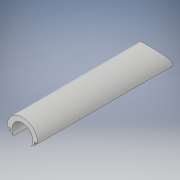
# Autodesk Inventor part: drone motor arm top
Saved by Autodesk Inventor 2019 (Build 230136000, 136)
## iProperties
Created: 2020-03-26
Part Number: drone motor arm top
Material: Generic
Document SubType Name: Modeling
Designer: Administrator
Density: 1 g/cm^3
Appearance: Default
Title: drone motor wrapper
Author: Administrator
Autodesk Inventor part; units mm, degrees
ref_plane "YZ Plane" through (0, 0, 0) normal (1, 0, 0) x (0, 1, 0)
ref_plane "Work Plane2" through (0.0017, -6.74, -2) normal (0, 1, 0) x (-1, 0, 0)
sketch "Sketch1" plane through (0.0017, -6.74, -2) normal (0, 1, 0) x (-1, 0, 0)
  line L0 (-2.7483, 0) -> (0, 0) construction
  line L1 (0, 0) -> (0.0017, 6)
  line L2 (1.7517, 6) -> (-1.7483, 6) construction
  arc A0 (-3.9294, 1.3826) -> (-4.2492, 3) centre (0.0008, 3) ccw construction
  arc A1 (-3.413, 0.4685) -> (3.4132, 0.4666) centre (0.0008, 3) ccw construction
  line L3 (5.1396, 2.9983) -> (6.2508, 2.9983)
  arc A2 (-6.2492, 3.0017) -> (6.2508, 2.9983) centre (0.0008, 3) ccw construction
  line L4 (5.7129, 2.1908) -> (5.1396, 2.1908) construction
  line L5 (5.1396, 2.1908) -> (5.1396, 2.9983) construction
  line L6 (-5.138, 3.0011) -> (-6.2492, 3.0017)
  line L7 (-5.7117, 2.194) -> (-5.1384, 2.1937) construction
  line L8 (-5.1384, 2.1937) -> (-5.138, 3.0011) construction
  line L9 (5.7129, 2.1908) -> (3.4132, 0.4666) construction
  line L10 (-5.7117, 2.194) -> (-3.413, 0.4685) construction
  line L11 (5.1396, 2.5258) -> (4.8896, 2.5258) construction
  line L12 (5.1396, 2.1908) -> (5.1396, 2.0408) construction
  line L13 (4.7148, 1.4425) -> (4.6248, 1.5625) construction
  line L14 (5.2628, 2.0408) -> (4.6248, 1.5625)
  line L15 (5.2628, 2.0408) -> (4.8896, 2.0408)
  line L16 (5.1396, 2.9983) -> (4.8896, 2.9983)
  line L17 (4.8896, 2.0408) -> (4.8896, 2.9983)
  line L18 (4.6248, 1.5625) -> (3.6609, 0.8398)
  arc A3 (3.6609, 0.8398) -> (4.2508, 2.9983) centre (0.0008, 3) ccw
  line L19 (-5.2617, 2.0437) -> (-4.624, 1.5651)
  line L20 (-5.2617, 2.0437) -> (-4.8885, 2.0435)
  line L21 (-5.138, 3.0011) -> (-4.888, 3.001)
  line L22 (-4.8885, 2.0435) -> (-4.888, 3.001)
  line L23 (-4.624, 1.5651) -> (-3.6604, 0.8418)
  arc A4 (-4.2492, 3.0006) -> (-3.6604, 0.8418) centre (0.0008, 3) ccw
  arc A5 (4.2508, 2.9983) -> (-4.2492, 3.0006) centre (0.0008, 3) ccw
  arc A6 (-6.2492, 3.0017) -> (6.2508, 2.9983) centre (0.0008, 3) ccw construction
  arc A7 (6.2508, 2.9983) -> (-6.2492, 3.0017) centre (0.0008, 3) ccw
  point P0 (0.0017, 2)
  point P1 (3.9302, 1.3805)
  dimension "d0" = 8.5
  dimension "d3" = 12.5
  constraints: 48 end point, 18 point on circle, 12 symmetric about line, 8 centre point, 7 concentric, 5 horizontal, 2 midpoint, 2 perpendicular, 2 point on line, 2 vertical, 1 other
  measures "d0" diameter of A0
  measures "d3" distance of L6.end L3.end
extrude "Extrusion4" add sketch "Sketch1" against normal blind 50.8
ref_plane "Work Plane3" through (0, 0, -8) normal (0, 0, -1) x (-1, 0.0001, 0)
sketch "Sketch2" plane through (0, 0, -8) normal (0, 0, -1) x (-1, 0.0001, 0)
  circle A0 centre (0, 0) radius 6.74
  constraints: 1 centre point, 1 coincident
extrude "Extrusion5" add sketch "Sketch1" along normal blind 5
extrude "Extrusion6" cut sketch "Sketch2" against normal blind 100
sketch "Sketch3" plane through (4.8902, -57.54, 0.0435) normal (1, 0, 0.0006) x (0.0006, 0, -1)
  line L0 (-0.0029, 0) -> (1.199, 0) projected
  line L1 (1.199, 0) -> (1.2011, 10) construction
  line L2 (1.2011, 51.8817) -> (1.2011, 0) projected
  line L3 (1.2011, 10) -> (1.2011, 20)
  line L4 (1.2011, 20) -> (1.2011, 30) construction
  line L5 (1.2011, 30) -> (1.2011, 40)
  line L6 (1.2011, 40) -> (1.2011, 50) construction
  line L7 (-0.9574, 55.0191) -> (-0.9574, 0) projected
  line L8 (1.2011, 50) -> (-0.9574, 50)
  line L9 (-0.9574, 50) -> (-0.9574, 55.0191)
  line L10 (-0.9574, 55.0191) -> (1.2011, 55.0191)
  line L11 (1.2011, 55.0191) -> (1.2011, 50)
  line L12 (-0.9601, 52.8994) -> (-0.9601, 0) projected
  line L13 (1.2011, 40) -> (-0.9601, 40)
  line L14 (-0.9601, 40) -> (-0.9601, 30)
  line L15 (-0.9601, 30) -> (1.2011, 30)
  line L16 (1.2011, 30) -> (1.2011, 40)
  line L17 (1.2011, 20) -> (-0.9601, 20)
  line L18 (-0.9601, 20) -> (-0.9601, 10)
  line L19 (-0.9601, 10) -> (1.2011, 10)
  line L20 (1.2011, 10) -> (1.2011, 20)
  point P0 (0.0408, 57.54)
  dimension "d27" = 10
  dimension "d28" = 10
  dimension "d29" = 10
  dimension "d30" = 10
  dimension "d31" = 10
  constraints: 34 end point, 7 point on line, 6 parallel, 3 horizontal, 3 perpendicular
  measures "d27" distance of L0.end L1.end
  measures "d28" distance of L1.end L3.end
  measures "d29" distance of L3.end L4.end
  measures "d30" distance of L4.end L5.end
  measures "d31" distance of L5.end L6.end
extrude "Extrusion7" cut sketch "Sketch3" along normal mid plane 100 contours L2 L8 L7 L10 L11 | L2 L15 L7 L13 | L7 L15 L12 L13 | L2 L19 L7 L17 | L7 L19 L12 L17
body "Solid1"
body "Solid5"
